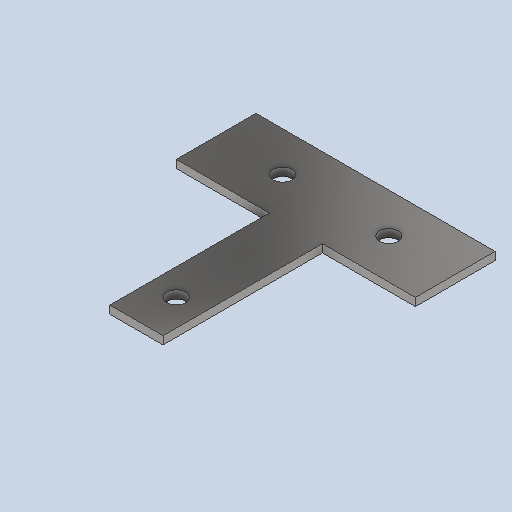
# Autodesk Inventor part: HCMUTE-CDT23-OP_TAMLOT
Saved by Autodesk Inventor 2023 (Build 270158000, 158)
## iProperties
Created: 2023-11-19
Part Number: HCMUTE-CDT23-OP_TAMLOT
Material: Stainless Steel
Document SubType Name: Sheet Metal
Designer: havie
Density: 8 g/cm^3
Sheet Metal Rule: Default_mm
Appearance: Steel - Polished
Author: havie
Autodesk Inventor part; units mm, degrees
ref_plane "YZ Plane" through (0, 0, 0) normal (1, 0, 0) x (0, 1, 0)
ref_plane "XZ Plane" through (0, 0, 0) normal (0, 1, 0) x (-1, 0, 0)
ref_plane "XY Plane" through (0, 0, 0) normal (0, 0, 1) x (1, 0, 0)
sketch "Sketch1" plane through (0, 0, 0) normal (0, 1, 0) x (-1, 0, 0)
  line L0 (-10, 0) -> (-10, 60)
  line L1 (-10, 60) -> (10, 60)
  line L2 (10, 60) -> (10, 0)
  line L3 (10, 0) -> (45, 0)
  line L4 (45, 0) -> (45, -30)
  line L5 (45, -30) -> (-45, -30)
  line L6 (-45, -30) -> (-45, 0)
  line L7 (-45, 0) -> (-10, 0)
  point P0 (0, 0)
  point P1 (0, 60)
  dimension "d0" = 20
  dimension "d1" = 30
  dimension "d2" = 60
  dimension "d3" = 90
  measures "d0" distance of L0.end L1.end
  measures "d1" distance of L5.end L6.end
  measures "d2" distance of L0.start L0.end
  measures "d3" distance of L4.end L5.end
extrude "Plate1" add sketch "Sketch1" along normal mid plane 3
sketch "Sketch2" plane through (0, 1.5, 0) normal (0, 1, 0) x (1, 0, 0)
  line L0 (10, -60) -> (-10, -60) projected
  line L1 (45, 30) -> (45, 0) projected
  line L2 (-45, 0) -> (-45, 30) projected
  point P0 (0, 0)
  point P1 (0, -45)
  point P2 (20, 15)
  point P3 (-20, 15)
  point P4 (-45, 15)
  dimension "d5" = 15
  dimension "d6" = 25
  dimension "d7" = 25
  constraints: 2 horizontal alignment, 1 midpoint, 1 vertical alignment
  measures "d5" distance from line of L0 point (0, -45)
  measures "d6" distance from line of L1 point (20, 15)
  measures "d7" distance from line of L2 point (-20, 15)
hole "Hole1" at (0, 1.5, 45) at (20, 1.5, -15) at (-20, 1.5, -15) direction (0, -1, 0) diameter 7 depth 3
equation "\"d6\" = d7"
equation "\"d13\" = Thickness"
equation "\"d4\" = Thickness"
equation "\"BendRadius\" = Thickness"
equation "\"BendReliefWidth\" = Thickness"
equation "\"BendReliefDepth\" = 0.5 * Thickness"
equation "\"CornerReliefSize\" = 4 * Thickness"
equation "\"MinimumRemnant\" = 2 * Thickness"
equation "\"TransitionRadius\" = BendRadius"
equation "\"JacobiRadiusSize\" = BendRadius"
equation "\"GapSize\" = Thickness"
equation "\"Thickness\" = 3"
body "Solid1"
